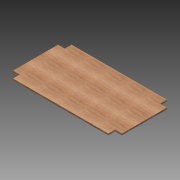
# Autodesk Inventor part: cart shelf
Saved by Autodesk Inventor 2013 (Build 170138000, 138)
## iProperties
Created: 2013-01-03
Part Number: cart shelf
Material: Wood (Birch)
Document SubType Name: Modeling
Designer: Arpan
Density: 1 g/cm^3
Author: Arpan
Autodesk Inventor part; units mm, degrees
ref_plane "YZ Plane" through (0, 0, 0) normal (1, 0, 0) x (0, 1, 0)
ref_plane "XZ Plane" through (0, 0, 0) normal (0, 1, 0) x (-1, 0, 0)
ref_plane "XY Plane" through (0, 0, 0) normal (0, 0, 1) x (1, 0, 0)
sketch "Sketch1" plane through (0, 0, 0) normal (0, 1, 0) x (-1, 0, 0)
  line L0 (-82.55, -82.55) -> (-1238.25, -82.55)
  line L1 (-1320.8, 0) -> (-1320.8, 546.1)
  line L2 (-1238.25, 628.65) -> (-82.55, 628.65)
  line L3 (0, 546.1) -> (0, 0)
  line L4 (-1238.25, 628.65) -> (-1238.25, 546.1)
  line L5 (-1238.25, 546.1) -> (-1320.8, 546.1)
  line L6 (-1238.25, -82.55) -> (-1238.25, 0)
  line L7 (-1238.25, 0) -> (-1320.8, 0)
  line L8 (-82.55, 628.65) -> (-82.55, 546.1)
  line L9 (-82.55, 546.1) -> (0, 546.1)
  line L10 (-82.55, -82.55) -> (-82.55, 0)
  line L11 (-82.55, 0) -> (0, 0)
  point P0 (0, 0)
  dimension "d2" = 82.55
  dimension "d3" = 82.55
  dimension "d4" = 82.55
  dimension "d5" = 82.55
  dimension "d6" = 82.55
  dimension "d7" = 82.55
  dimension "d8" = 82.55
  dimension "d9" = 82.55
  dimension "d10" = 90
  dimension "d11" = 90
  dimension "d12" = 90
  dimension "d13" = 90
  dimension "d14" = 90
  dimension "d15" = 90
  dimension "d16" = 90
  dimension "d17" = 90
  dimension "d20" = 711.2
  constraints: 24 end point, 2 parallel, 1 horizontal, 1 perpendicular
  measures "d2" distance of L2.start L4.end
  measures "d3" distance of L1.end L4.end
  measures "d4" distance of L1.start L6.end
  measures "d5" distance of L0.end L6.end
  measures "d6" distance of L3.start L8.end
  measures "d7" distance of L2.end L8.end
  measures "d8" distance of L3.end L10.end
  measures "d9" distance of L0.start L10.end
  measures "d10" angle of L8 L2
  measures "d11" angle of L3 L9
  measures "d12" angle of L1 L5
  measures "d13" angle of L2 L4
  measures "d14" angle of L6 L7
  measures "d15" angle of L0 L6
  measures "d16" angle of L0 L10
  measures "d17" angle of L3 L11
  measures "d20" distance between parallel lines of L2 L0
extrude "Extrusion1" add sketch "Sketch1" along normal blind 19.05
body "Solid1"
